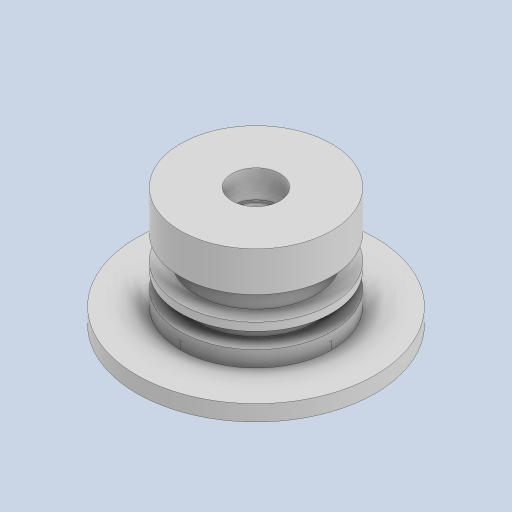
# Autodesk Inventor part: диск
Saved by Autodesk Inventor 2024.2 (Build 282272000, 272)
## iProperties
Created: 2025-11-25
Part Number: диск
Material: Типовые
Document SubType Name: Modeling
Designer: katya_notebook
Density: 1 g/cm^3
Appearance: По умолчанию
Author: katya_notebook
Autodesk Inventor part; units mm, degrees
ref_plane "YZ Plane" through (0, 0, 0) normal (1, 0, 0) x (0, 1, 0)
ref_plane "XZ Plane" through (0, 0, 0) normal (0, 1, 0) x (-1, 0, 0)
ref_plane "XY Plane" through (0, 0, 0) normal (0, 0, 1) x (1, 0, 0)
sketch "Эскиз1" plane through (0, 0, 0) normal (0, 1, 0) x (-1, 0, 0)
  circle A0 centre (0, 0) radius 9.5
  dimension "d0" = 19
  constraints: 1 centre point, 1 coincident
  measures "d0" diameter of A0
extrude "Выдавливание1" add sketch "Эскиз1" along normal blind 5
sketch "Эскиз2" plane through (0, 0, 0) normal (0, -1, 0) x (1, 0, 0)
  circle A0 centre (0, 0) radius 7.5
  dimension "d3" = 15
  constraints: 1 centre point, 1 coincident
  measures "d3" diameter of A0
extrude "Выдавливание2" add sketch "Эскиз2" along normal blind 3
sketch "Эскиз3" plane through (0, -3, 0) normal (0, -1, 0) x (1, 0, 0)
  circle A0 centre (0, 0) radius 9.5
  dimension "d15" = 19
  constraints: 1 centre point, 1 coincident
  measures "d15" diameter of A0
extrude "Выдавливание3" add sketch "Эскиз3" along normal blind 1
sketch "Эскиз4" plane through (0, -4, 0) normal (0, -1, 0) x (1, 0, 0)
  circle A0 centre (0, 0) radius 7.5
  dimension "d17" = 15
  constraints: 1 centre point, 1 coincident
  measures "d17" diameter of A0
extrude "Выдавливание4" add sketch "Эскиз4" along normal blind 2
sketch "Эскиз5" plane through (0, -6, 0) normal (0, -1, 0) x (1, 0, 0)
  circle A0 centre (0, 0) radius 9.5
  dimension "d16" = 19
  constraints: 1 centre point, 1 coincident
  measures "d16" diameter of A0
extrude "Выдавливание5" add sketch "Эскиз5" along normal blind 2
sketch "Эскиз8" plane through (0, -8, 0) normal (0, -1, 0) x (1, 0, 0)
  circle A0 centre (0, 0) radius 15
  dimension "d21" = 30
  constraints: 1 centre point, 1 coincident
  measures "d21" diameter of A0
extrude "Выдавливание8" add sketch "Эскиз8" along normal blind 2
sketch "Эскиз6" plane through (0, 5, 0) normal (0, 1, 0) x (1, 0, 0)
  circle A0 centre (0, 0) radius 2.6
  dimension "d12" = 5.2
  constraints: 1 centre point, 1 coincident
  measures "d12" diameter of A0
extrude "Выдавливание6" cut sketch "Эскиз6" against normal blind 27
sketch "Эскиз7" plane through (0, 5, 0) normal (0, 1, 0) x (1, 0, 0)
  circle A0 centre (0, 0) radius 3
  dimension "d18" = 6
  constraints: 1 centre point, 1 coincident
  measures "d18" diameter of A0
extrude "Выдавливание7" cut sketch "Эскиз7" against normal blind 3.5
sketch "Эскиз9" plane through (0, -10, 0) normal (0, -1, 0) x (1, 0, 0)
  circle A0 centre (0, 8) radius 1.5
  circle A1 centre (-8, 0) radius 1.5
  circle A2 centre (0, -8) radius 1.5
  circle A3 centre (8, 0) radius 1.5
  circle A4 centre (-8, 0) radius 1.5
  circle A5 centre (0, 8) radius 1.5
  circle A6 centre (8, 0) radius 1.5
  circle A7 centre (0, -8) radius 1.5
  point P0 (0, 0)
  point P1 (0, 0)
  constraints: 8 centre point, 4 coincident, 4 concentric
extrude "Выдавливание9" cut sketch "Эскиз9" against normal blind 3
thread "Резьба1" size "M3x0.5" class "6H" standard "ANSI Metric M Profile" full length
thread "Резьба2" size "M3x0.5" class "6H" standard "ANSI Metric M Profile" full length
thread "Резьба3" size "M3x0.5" class "6H" standard "ANSI Metric M Profile" full length
thread "Резьба4" size "M3x0.5" class "6H" standard "ANSI Metric M Profile" full length
